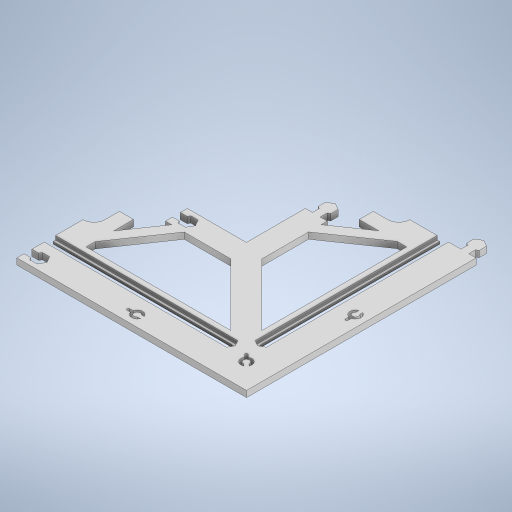
# Autodesk Inventor part: Vnejsi_ram
Saved by Autodesk Inventor 2024.2 (Build 282272000, 272)
## iProperties
Created: 2025-05-26
Part Number: Vnejsi_ram
Material: Všeobecné
Document SubType Name: Modeling
Designer: Elite
Density: 1 g/cm^3
Appearance: Výchozí
Author: Elite
Autodesk Inventor part; units mm, degrees
ref_plane "YZ Plane" through (0, 0, 0) normal (1, 0, 0) x (0, 1, 0)
ref_plane "XZ Plane" through (0, 0, 0) normal (0, 1, 0) x (-1, 0, 0)
ref_plane "XY Plane" through (0, 0, 0) normal (0, 0, 1) x (1, 0, 0)
sketch "Náčrt1" plane through (0, 0, 0) normal (0, 0, 1) x (1, 0, 0)
  line L0 (-41.907, -49.2472) -> (-39.5976, -53.2472)
  line L1 (-39.5976, -53.2472) -> (-41.907, -57.2472)
  line L2 (-41.907, -57.2472) -> (-46.5258, -57.2472)
  line L3 (-46.5258, -49.2472) -> (-41.907, -49.2472)
  line L4 (7.4742, -57.2472) -> (12.093, -57.2472)
  line L5 (12.093, -57.2472) -> (14.4024, -53.2472)
  line L6 (14.4024, -53.2472) -> (12.093, -49.2472)
  line L7 (12.093, -49.2472) -> (7.4742, -49.2472)
  line L8 (6.6082, -50.7472) -> (2.2836, -50.7472)
  line L9 (7.4742, -49.2472) -> (6.6082, -50.7472)
  line L10 (2.2836, -55.7472) -> (6.6082, -55.7472)
  line L11 (6.6082, -55.7472) -> (7.4742, -57.2472)
  line L12 (2.2836, -60.2472) -> (2.2836, -55.7472)
  line L13 (2.2836, -50.7472) -> (2.2836, -46.2472)
  line L14 (-17.7164, -60.2472) -> (2.2836, -60.2472)
  line L15 (2.2836, -46.2472) -> (-17.7164, -46.2472)
  line L16 (50.8236, 1.1022) -> (46.8236, 3.4116)
  line L17 (46.8236, 3.4116) -> (50.8236, 1.1022)
  line L18 (42.8236, 1.1022) -> (46.8236, 3.4116)
  line L19 (49.3236, -8.7072) -> (49.3236, -4.3826)
  line L20 (42.8236, -3.5166) -> (44.3236, -4.3826)
  line L21 (53.8236, -8.7072) -> (49.3236, -8.7072)
  line L22 (49.3236, -8.7072) -> (53.8236, -8.7072)
  line L23 (42.8236, 1.1022) -> (42.8236, -3.5166)
  line L24 (42.8236, -3.5166) -> (42.8236, 1.1022)
  line L25 (44.3236, -4.3826) -> (42.8236, -3.5166)
  line L26 (44.3236, -4.3826) -> (44.3236, -8.7072)
  line L27 (44.3236, -8.7072) -> (39.8236, -8.7072)
  line L28 (39.8236, -8.7072) -> (44.3236, -8.7072)
  line L29 (44.3236, -8.7072) -> (44.3236, -4.3826)
  line L30 (46.8236, 3.4116) -> (42.8236, 1.1022)
  line L31 (50.8236, -3.5166) -> (50.8236, 1.1022)
  line L32 (50.8236, 1.1022) -> (50.8236, -3.5166)
  line L33 (49.3236, -4.3826) -> (50.8236, -3.5166)
  line L34 (50.8236, -3.5166) -> (49.3236, -4.3826)
  line L35 (49.3236, -4.3826) -> (49.3236, -8.7072)
  line L36 (53.8236, 11.2928) -> (53.8236, -8.7072)
  line L37 (53.8236, -8.7072) -> (53.8236, 11.2928)
  line L38 (39.8236, -8.7072) -> (39.8236, 11.2928)
  line L39 (39.8236, 11.2928) -> (39.8236, -8.7072)
  line L40 (2.2836, -60.2472) -> (53.8236, -60.2472)
  line L41 (53.8236, -60.2472) -> (53.8236, -8.7072)
  line L42 (39.8236, -8.7072) -> (39.8236, -46.2472)
  line L43 (39.8236, -46.2472) -> (2.2836, -46.2472)
  arc A0 (-31.7164, -78.7074) -> (-17.7164, -78.7074) centre (-24.7164, -78.7074) ccw
  arc A1 (72.2839, 11.2928) -> (72.2839, 25.2928) centre (72.2839, 18.2928) ccw
  line L44 (53.8236, 11.2928) -> (72.2839, 11.2928)
  line L45 (72.2839, 25.2928) -> (53.8236, 25.2928)
  line L46 (-1.0283, -5.3953) -> (2.0296, -2.3374)
  line L47 (2.0296, -2.3374) -> (-1.0283, -5.3953)
  line L48 (2.0296, -2.3374) -> (3.7027, -2.7856)
  line L49 (3.7027, -2.7856) -> (2.0296, -2.3374)
  line L50 (3.5679, -9.9915) -> (-1.0283, -5.3953)
  line L51 (-1.0283, -5.3953) -> (3.5679, -9.9915)
  line L52 (-48.4045, -5.3953) -> (-53.0006, -9.9915)
  line L53 (-53.0006, -9.9915) -> (-48.4045, -5.3953)
  line L54 (-45.3465, -8.4532) -> (-48.4045, -5.3953)
  line L55 (-48.4045, -5.3953) -> (-45.3465, -8.4532)
  line L56 (-45.7948, -10.1263) -> (-45.3465, -8.4532)
  line L57 (-45.7948, -10.1263) -> (-42.5288, -13.3922)
  line L58 (-45.3465, -8.4532) -> (-45.7948, -10.1263)
  line L59 (-41.811, -4.9177) -> (-40.1379, -4.4694)
  line L60 (-40.1379, -4.4694) -> (-41.811, -4.9177)
  line L61 (-42.5288, -13.3922) -> (-45.7948, -10.1263)
  line L62 (-40.1379, -4.4694) -> (-36.872, -7.7354)
  line L63 (-36.872, -7.7354) -> (-40.1379, -4.4694)
  line L64 (-42.5288, -13.3922) -> (-38.0674, -12.1968)
  line L65 (-38.0674, -12.1968) -> (-36.872, -7.7354)
  line L66 (-36.872, -7.7354) -> (-38.0674, -12.1968)
  line L67 (-38.0674, -12.1968) -> (-42.5288, -13.3922)
  line L68 (-44.8689, -1.8598) -> (-41.811, -4.9177)
  line L69 (-41.811, -4.9177) -> (-44.8689, -1.8598)
  line L70 (-24.7164, -80.7891) -> (-28.3164, -78.7107)
  arc A2 (-26.7914, -76.5379) -> (-22.6414, -76.4898) centre (-24.715, -76.6291) ccw
  line L71 (-24.7164, -80.7891) -> (-28.3164, -78.7107)
  arc A3 (-31.7164, -78.7074) -> (-17.7164, -78.7074) centre (-24.7164, -78.7074) ccw
  arc A4 (-26.7914, -76.5379) -> (-22.6414, -76.4898) centre (-24.715, -76.6291) ccw
  line L72 (-21.1164, -78.7107) -> (-24.7164, -80.7891)
  line L73 (-21.1164, -78.7107) -> (-24.7164, -80.7891)
  line L74 (-31.7164, -60.2472) -> (-31.7164, -78.7074)
  line L75 (-31.7164, -78.7074) -> (-31.7164, -60.2472)
  line L76 (-17.7164, -60.2472) -> (-17.7164, -78.7074)
  line L77 (-17.7164, -78.7074) -> (-17.7164, -60.2472)
  line L78 (-41.907, -57.2472) -> (-39.5976, -53.2472)
  line L79 (-51.7164, -55.7472) -> (-47.3918, -55.7472)
  line L80 (-46.5258, -49.2472) -> (-47.3918, -50.7472)
  line L81 (-31.7164, -60.2472) -> (-51.7164, -60.2472)
  line L82 (-51.7164, -60.2472) -> (-31.7164, -60.2472)
  line L83 (-51.7164, -60.2472) -> (-51.7164, -55.7472)
  line L84 (-51.7164, -55.7472) -> (-51.7164, -60.2472)
  line L85 (-41.907, -49.2472) -> (-46.5258, -49.2472)
  line L86 (-47.3918, -50.7472) -> (-46.5258, -49.2472)
  line L87 (-51.7164, -46.2472) -> (-31.7164, -46.2472)
  line L88 (-31.7164, -46.2472) -> (-51.7164, -46.2472)
  line L89 (-47.3918, -50.7472) -> (-51.7164, -50.7472)
  line L90 (-51.7164, -50.7472) -> (-51.7164, -46.2472)
  line L91 (-51.7164, -46.2472) -> (-51.7164, -50.7472)
  line L92 (-51.7164, -50.7472) -> (-47.3918, -50.7472)
  line L93 (-26.7914, -29.9633) -> (-26.7914, -76.5379)
  line L94 (2.2836, -46.2472) -> (2.2836, -50.7472)
  line L95 (2.2836, -50.7472) -> (6.6082, -50.7472)
  line L96 (6.6082, -55.7472) -> (2.2836, -55.7472)
  line L97 (-24.7164, -25.7052) -> (-21.1164, -27.7837)
  line L98 (-28.3164, -27.7837) -> (-24.7164, -25.7052)
  line L99 (-17.7164, -21.0899) -> (-17.7164, -46.2472)
  arc A5 (-22.6414, -29.8845) -> (-26.7914, -29.9633) centre (-24.7175, -29.8628) ccw
  arc A6 (-53.0006, -9.9915) -> (-31.7164, -21.0899) centre (-24.7164, 18.2928) ccw
  arc A7 (-53.0006, -9.9915) -> (-31.7164, -21.0899) centre (-24.7164, 18.2928) ccw
  line L100 (-48.4045, -5.3953) -> (-45.3465, -8.4532)
  line L101 (-45.3465, -8.4532) -> (-48.4045, -5.3953)
  line L102 (-42.5288, -13.3922) -> (-38.0674, -12.1968)
  line L103 (-38.0674, -12.1968) -> (-42.5288, -13.3922)
  line L104 (-45.7948, -10.1263) -> (-42.5288, -13.3922)
  line L105 (-42.5288, -13.3922) -> (-45.7948, -10.1263)
  line L106 (-38.0674, -12.1968) -> (-36.872, -7.7354)
  line L107 (-36.872, -7.7354) -> (-38.0674, -12.1968)
  line L108 (-45.3465, -8.4532) -> (-45.7948, -10.1263)
  line L109 (-45.7948, -10.1263) -> (-45.3465, -8.4532)
  line L110 (-40.1379, -4.4694) -> (-36.872, -7.7354)
  line L111 (-36.872, -7.7354) -> (-40.1379, -4.4694)
  line L112 (-53.0006, -9.9915) -> (-48.4045, -5.3953)
  line L113 (-48.4045, -5.3953) -> (-53.0006, -9.9915)
  arc A8 (-17.7164, -21.0899) -> (3.5679, -9.9915) centre (-24.7164, 18.2928) ccw
  arc A9 (-17.7164, -21.0899) -> (3.5679, -9.9915) centre (-24.7164, 18.2928) ccw
  line L114 (-1.0283, -5.3953) -> (3.5679, -9.9915)
  line L115 (3.5679, -9.9915) -> (-1.0283, -5.3953)
  line L116 (2.0296, -2.3374) -> (-1.0283, -5.3953)
  line L117 (-1.0283, -5.3953) -> (2.0296, -2.3374)
  line L118 (3.7027, -2.7856) -> (2.0296, -2.3374)
  line L119 (2.0296, -2.3374) -> (3.7027, -2.7856)
  line L120 (-24.7164, -25.7052) -> (-21.1164, -27.7837)
  arc A10 (-22.6414, -29.8845) -> (-26.7914, -29.9633) centre (-24.7175, -29.8628) ccw
  line L121 (-28.3164, -27.7837) -> (-24.7164, -25.7052)
  line L122 (-17.7164, -46.2472) -> (-17.7164, -21.0899)
  line L123 (-31.7164, -46.2472) -> (-31.7164, -21.0899)
  line L124 (-31.7164, -21.0899) -> (-31.7164, -46.2472)
  line L125 (-39.5976, -53.2472) -> (-41.907, -49.2472)
  line L126 (-22.6414, -76.4898) -> (-22.6414, -29.8845)
  line L127 (-22.6414, -76.4898) -> (-22.6414, -29.8845)
  line L128 (-26.7914, -29.9633) -> (-26.7914, -76.5379)
  line L129 (-21.1164, -27.7837) -> (-21.1164, -78.7107)
  line L130 (-21.1164, -27.7837) -> (-21.1164, -78.7107)
  line L131 (-28.3164, -78.7107) -> (-28.3164, -27.7837)
  line L132 (-28.3164, -78.7107) -> (-28.3164, -27.7837)
  line L133 (-46.5258, -57.2472) -> (-41.907, -57.2472)
  line L134 (-47.3918, -55.7472) -> (-46.5258, -57.2472)
  line L135 (-46.5258, -57.2472) -> (-47.3918, -55.7472)
  line L136 (-47.3918, -55.7472) -> (-51.7164, -55.7472)
  line L137 (-40.1379, -4.4694) -> (-41.811, -4.9177)
  line L138 (-41.811, -4.9177) -> (-40.1379, -4.4694)
  line L139 (-41.811, -4.9177) -> (-44.8689, -1.8598)
  line L140 (-44.8689, -1.8598) -> (-41.811, -4.9177)
  line L141 (2.2836, -55.7472) -> (2.2836, -60.2472)
  line L142 (2.2836, -60.2472) -> (-17.7164, -60.2472)
  line L143 (-17.7164, -46.2472) -> (2.2836, -46.2472)
  line L144 (74.3655, 18.2928) -> (72.2871, 14.6928)
  arc A11 (70.1143, 16.2178) -> (70.0662, 20.3678) centre (70.2055, 18.2941) ccw
  line L145 (74.3655, 18.2928) -> (72.2871, 14.6928)
  arc A12 (72.2839, 11.2928) -> (72.2839, 25.2928) centre (72.2839, 18.2928) ccw
  arc A13 (70.1143, 16.2178) -> (70.0662, 20.3678) centre (70.2055, 18.2941) ccw
  line L146 (72.2871, 21.8928) -> (74.3655, 18.2928)
  line L147 (72.2871, 21.8928) -> (74.3655, 18.2928)
  line L148 (72.2839, 11.2928) -> (53.8236, 11.2928)
  line L149 (53.8236, 25.2928) -> (72.2839, 25.2928)
  line L150 (23.5397, 16.2178) -> (70.1143, 16.2178)
  line L151 (39.8236, 45.2928) -> (44.3236, 45.2928)
  line L152 (44.3236, 45.2928) -> (39.8236, 45.2928)
  line L153 (44.3236, 45.2928) -> (44.3236, 49.6174)
  line L154 (44.3236, 49.6174) -> (44.3236, 45.2928)
  line L155 (44.3236, 49.6174) -> (42.8236, 50.4834)
  line L156 (42.8236, 50.4834) -> (44.3236, 49.6174)
  line L157 (42.8236, 50.4834) -> (42.8236, 55.1022)
  line L158 (42.8236, 55.1022) -> (42.8236, 50.4834)
  line L159 (42.8236, 55.1022) -> (46.8236, 57.4116)
  line L160 (49.3236, 49.6174) -> (49.3236, 45.2928)
  line L161 (49.3236, 45.2928) -> (49.3236, 49.6174)
  line L162 (50.8236, 50.4834) -> (49.3236, 49.6174)
  line L163 (49.3236, 49.6174) -> (50.8236, 50.4834)
  line L164 (50.8236, 55.1022) -> (50.8236, 50.4834)
  line L165 (50.8236, 50.4834) -> (50.8236, 55.1022)
  line L166 (46.8236, 57.4116) -> (50.8236, 55.1022)
  line L167 (50.8236, 55.1022) -> (46.8236, 57.4116)
  line L168 (46.8236, 57.4116) -> (42.8236, 55.1022)
  line L169 (19.2816, 18.2928) -> (21.3601, 21.8928)
  line L170 (21.3601, 14.6928) -> (19.2816, 18.2928)
  line L171 (14.6664, 25.2928) -> (39.8236, 25.2928)
  arc A14 (23.4609, 20.3678) -> (23.5397, 16.2178) centre (23.4392, 18.2916) ccw
  arc A15 (3.5679, -9.9915) -> (14.6664, 11.2928) centre (-24.7164, 18.2928) ccw
  arc A16 (3.5679, -9.9915) -> (14.6664, 11.2928) centre (-24.7164, 18.2928) ccw
  line L172 (6.9687, 0.4803) -> (5.7732, 4.9418)
  line L173 (5.7732, 4.9418) -> (6.9687, 0.4803)
  line L174 (3.7027, -2.7856) -> (6.9687, 0.4803)
  line L175 (6.9687, 0.4803) -> (3.7027, -2.7856)
  line L176 (5.7732, 4.9418) -> (1.3118, 6.1372)
  line L177 (1.3118, 6.1372) -> (5.7732, 4.9418)
  line L178 (-1.9542, 2.8712) -> (1.3118, 6.1372)
  line L179 (1.3118, 6.1372) -> (-1.9542, 2.8712)
  arc A17 (14.6664, 25.2928) -> (3.5679, 46.5771) centre (-24.7164, 18.2928) ccw
  arc A18 (14.6664, 25.2928) -> (3.5679, 46.5771) centre (-24.7164, 18.2928) ccw
  line L180 (-1.0283, 41.9809) -> (3.5679, 46.5771)
  line L181 (3.5679, 46.5771) -> (-1.0283, 41.9809)
  line L182 (-4.0862, 45.0388) -> (-1.0283, 41.9809)
  line L183 (-1.0283, 41.9809) -> (-4.0862, 45.0388)
  line L184 (-3.6379, 46.7118) -> (-4.0862, 45.0388)
  line L185 (-3.6379, 46.7118) -> (-6.9039, 49.9778)
  line L186 (-4.0862, 45.0388) -> (-3.6379, 46.7118)
  line L187 (-7.6218, 41.5033) -> (-9.2948, 41.055)
  line L188 (-9.2948, 41.055) -> (-7.6218, 41.5033)
  line L189 (-6.9039, 49.9778) -> (-3.6379, 46.7118)
  line L190 (-9.2948, 41.055) -> (-12.5608, 44.321)
  line L191 (-12.5608, 44.321) -> (-9.2948, 41.055)
  line L192 (-6.9039, 49.9778) -> (-11.3654, 48.7824)
  line L193 (-11.3654, 48.7824) -> (-12.5608, 44.321)
  line L194 (-12.5608, 44.321) -> (-11.3654, 48.7824)
  line L195 (-11.3654, 48.7824) -> (-6.9039, 49.9778)
  line L196 (19.2816, 18.2928) -> (21.3601, 21.8928)
  arc A19 (23.4609, 20.3678) -> (23.5397, 16.2178) centre (23.4392, 18.2916) ccw
  line L197 (21.3601, 14.6928) -> (19.2816, 18.2928)
  line L198 (39.8236, 25.2928) -> (14.6664, 25.2928)
  line L199 (39.8236, 11.2928) -> (14.6664, 11.2928)
  line L200 (14.6664, 11.2928) -> (39.8236, 11.2928)
  line L201 (70.0662, 20.3678) -> (23.4609, 20.3678)
  line L202 (70.0662, 20.3678) -> (23.4609, 20.3678)
  line L203 (23.5397, 16.2178) -> (70.1143, 16.2178)
  line L204 (21.3601, 21.8928) -> (72.2871, 21.8928)
  line L205 (21.3601, 21.8928) -> (72.2871, 21.8928)
  line L206 (72.2871, 14.6928) -> (21.3601, 14.6928)
  line L207 (72.2871, 14.6928) -> (21.3601, 14.6928)
  line L208 (-1.9542, 2.8712) -> (-1.5059, 1.1982)
  line L209 (-1.5059, 1.1982) -> (-1.9542, 2.8712)
  line L210 (-1.5059, 1.1982) -> (-4.5638, -1.8598)
  line L211 (-4.5638, -1.8598) -> (-1.5059, 1.1982)
  line L212 (-4.5638, 38.4453) -> (-7.6218, 41.5033)
  line L213 (-7.6218, 41.5033) -> (-4.5638, 38.4453)
  line L214 (-4.5638, -1.8598) -> (-21.1808, 14.7573)
  line L215 (-21.1808, 14.7573) -> (-4.5638, -1.8598)
  arc A20 (-21.1808, 14.7573) -> (-21.1808, 21.8283) centre (-24.7164, 18.2928) ccw
  arc A21 (-21.1808, 14.7573) -> (-21.1808, 21.8283) centre (-24.7164, 18.2928) ccw
  line L216 (-4.5638, 38.4453) -> (-21.1808, 21.8283)
  line L217 (-21.1808, 21.8283) -> (-4.5638, 38.4453)
  line L218 (39.8236, 45.2928) -> (39.8236, 25.2928)
  line L219 (53.8236, 45.2928) -> (49.3236, 45.2928)
  line L220 (53.8236, 25.2928) -> (53.8236, 45.2928)
  line L221 (49.3236, 45.2928) -> (53.8236, 45.2928)
  line L222 (53.8236, 45.2928) -> (53.8236, 25.2928)
  line L223 (39.8236, 25.2928) -> (39.8236, 45.2928)
  line L224 (-24.7164, 117.3747) -> (-21.1164, 115.2962)
  arc A22 (-22.6414, 113.1234) -> (-26.7914, 113.0754) centre (-24.7177, 113.2147) ccw
  line L225 (-24.7164, 117.3747) -> (-21.1164, 115.2962)
  arc A23 (-17.7164, 115.293) -> (-31.7164, 115.293) centre (-24.7164, 115.293) ccw
  arc A24 (-17.7164, 115.293) -> (-31.7164, 115.293) centre (-24.7164, 115.293) ccw
  arc A25 (-22.6414, 113.1234) -> (-26.7914, 113.0754) centre (-24.7177, 113.2147) ccw
  line L226 (-28.3164, 115.2962) -> (-24.7164, 117.3747)
  line L227 (-28.3164, 115.2962) -> (-24.7164, 117.3747)
  line L228 (-17.7164, 96.8328) -> (-17.7164, 115.293)
  line L229 (-17.7164, 115.293) -> (-17.7164, 96.8328)
  line L230 (-31.7164, 96.8328) -> (-31.7164, 115.293)
  line L231 (-31.7164, 115.293) -> (-31.7164, 96.8328)
  line L232 (-7.5258, 93.8328) -> (-9.8352, 89.8328)
  line L233 (-9.8352, 89.8328) -> (-7.5258, 93.8328)
  line L234 (-7.5258, 85.8328) -> (-9.8352, 89.8328)
  line L235 (2.2836, 92.3328) -> (-2.0409, 92.3328)
  line L236 (-2.907, 85.8328) -> (-2.0409, 87.3328)
  line L237 (-17.7164, 96.8328) -> (2.2836, 96.8328)
  line L238 (2.2836, 96.8328) -> (-17.7164, 96.8328)
  line L239 (2.2836, 96.8328) -> (2.2836, 92.3328)
  line L240 (2.2836, 92.3328) -> (2.2836, 96.8328)
  line L241 (-7.5258, 85.8328) -> (-2.907, 85.8328)
  line L242 (-2.907, 85.8328) -> (-7.5258, 85.8328)
  line L243 (-2.0409, 87.3328) -> (-2.907, 85.8328)
  line L244 (2.2836, 82.8328) -> (-17.7164, 82.8328)
  line L245 (-17.7164, 82.8328) -> (2.2836, 82.8328)
  line L246 (-2.0409, 87.3328) -> (2.2836, 87.3328)
  line L247 (2.2836, 87.3328) -> (2.2836, 82.8328)
  line L248 (2.2836, 82.8328) -> (2.2836, 87.3328)
  line L249 (2.2836, 87.3328) -> (-2.0409, 87.3328)
  line L250 (-22.6414, 66.5489) -> (-22.6414, 113.1234)
  line L251 (-51.7164, 82.8328) -> (-51.7164, 87.3328)
  line L252 (-51.7164, 87.3328) -> (-51.7164, 82.8328)
  line L253 (-51.7164, 87.3328) -> (-56.0409, 87.3328)
  line L254 (-56.0409, 87.3328) -> (-51.7164, 87.3328)
  line L255 (-56.0409, 87.3328) -> (-56.907, 85.8328)
  line L256 (-56.907, 85.8328) -> (-56.0409, 87.3328)
  line L257 (-56.907, 85.8328) -> (-61.5258, 85.8328)
  line L258 (-61.5258, 85.8328) -> (-56.907, 85.8328)
  line L259 (-61.5258, 85.8328) -> (-63.8352, 89.8328)
  line L260 (-56.0409, 92.3328) -> (-51.7164, 92.3328)
  line L261 (-51.7164, 92.3328) -> (-56.0409, 92.3328)
  line L262 (-56.907, 93.8328) -> (-56.0409, 92.3328)
  line L263 (-56.0409, 92.3328) -> (-56.907, 93.8328)
  line L264 (-61.5258, 93.8328) -> (-56.907, 93.8328)
  line L265 (-56.907, 93.8328) -> (-61.5258, 93.8328)
  line L266 (-63.8352, 89.8328) -> (-61.5258, 93.8328)
  line L267 (-61.5258, 93.8328) -> (-63.8352, 89.8328)
  line L268 (-63.8352, 89.8328) -> (-61.5258, 85.8328)
  line L269 (-24.7164, 62.2908) -> (-28.3164, 64.3693)
  line L270 (-21.1164, 64.3693) -> (-24.7164, 62.2908)
  line L271 (-31.7164, 57.6755) -> (-31.7164, 82.8328)
  arc A26 (-26.7914, 66.47) -> (-22.6414, 66.5489) centre (-24.7152, 66.4483) ccw
  arc A27 (3.5679, 46.5771) -> (-17.7164, 57.6755) centre (-24.7164, 18.2928) ccw
  arc A28 (3.5679, 46.5771) -> (-17.7164, 57.6755) centre (-24.7164, 18.2928) ccw
  line L272 (-1.0283, 41.9809) -> (-4.0862, 45.0388)
  line L273 (-4.0862, 45.0388) -> (-1.0283, 41.9809)
  line L274 (-6.9039, 49.9778) -> (-11.3654, 48.7824)
  line L275 (-11.3654, 48.7824) -> (-6.9039, 49.9778)
  line L276 (-3.6379, 46.7118) -> (-6.9039, 49.9778)
  line L277 (-6.9039, 49.9778) -> (-3.6379, 46.7118)
  line L278 (-11.3654, 48.7824) -> (-12.5608, 44.321)
  line L279 (-12.5608, 44.321) -> (-11.3654, 48.7824)
  line L280 (-4.0862, 45.0388) -> (-3.6379, 46.7118)
  line L281 (-3.6379, 46.7118) -> (-4.0862, 45.0388)
  line L282 (-9.2948, 41.055) -> (-12.5608, 44.321)
  line L283 (-12.5608, 44.321) -> (-9.2948, 41.055)
  line L284 (3.5679, 46.5771) -> (-1.0283, 41.9809)
  line L285 (-1.0283, 41.9809) -> (3.5679, 46.5771)
  arc A29 (-31.7164, 57.6755) -> (-53.0006, 46.5771) centre (-24.7164, 18.2928) ccw
  arc A30 (-31.7164, 57.6755) -> (-53.0006, 46.5771) centre (-24.7164, 18.2928) ccw
  line L286 (-48.4045, 41.9809) -> (-53.0006, 46.5771)
  line L287 (-53.0006, 46.5771) -> (-48.4045, 41.9809)
  line L288 (-51.4624, 38.9229) -> (-48.4045, 41.9809)
  line L289 (-48.4045, 41.9809) -> (-51.4624, 38.9229)
  line L290 (-53.1354, 39.3712) -> (-51.4624, 38.9229)
  line L291 (-53.1354, 39.3712) -> (-56.4014, 36.1052)
  line L292 (-51.4624, 38.9229) -> (-53.1354, 39.3712)
  line L293 (-47.9269, 35.3874) -> (-47.4786, 33.7144)
  line L294 (-47.4786, 33.7144) -> (-47.9269, 35.3874)
  line L295 (-56.4014, 36.1052) -> (-53.1354, 39.3712)
  line L296 (-47.4786, 33.7144) -> (-50.7446, 30.4484)
  line L297 (-50.7446, 30.4484) -> (-47.4786, 33.7144)
  line L298 (-56.4014, 36.1052) -> (-55.206, 31.6438)
  line L299 (-55.206, 31.6438) -> (-50.7446, 30.4484)
  line L300 (-50.7446, 30.4484) -> (-55.206, 31.6438)
  line L301 (-55.206, 31.6438) -> (-56.4014, 36.1052)
  line L302 (-24.7164, 62.2908) -> (-28.3164, 64.3693)
  arc A31 (-26.7914, 66.47) -> (-22.6414, 66.5489) centre (-24.7152, 66.4483) ccw
  line L303 (-21.1164, 64.3693) -> (-24.7164, 62.2908)
  line L304 (-31.7164, 82.8328) -> (-31.7164, 57.6755)
  line L305 (-17.7164, 82.8328) -> (-17.7164, 57.6755)
  line L306 (-17.7164, 57.6755) -> (-17.7164, 82.8328)
  line L307 (-9.8352, 89.8328) -> (-7.5258, 85.8328)
  line L308 (-26.7914, 113.0754) -> (-26.7914, 66.47)
  line L309 (-26.7914, 113.0754) -> (-26.7914, 66.47)
  line L310 (-22.6414, 66.5489) -> (-22.6414, 113.1234)
  line L311 (-28.3164, 64.3693) -> (-28.3164, 115.2962)
  line L312 (-28.3164, 64.3693) -> (-28.3164, 115.2962)
  line L313 (-21.1164, 115.2962) -> (-21.1164, 64.3693)
  line L314 (-21.1164, 115.2962) -> (-21.1164, 64.3693)
  line L315 (-2.907, 93.8328) -> (-7.5258, 93.8328)
  line L316 (-7.5258, 93.8328) -> (-2.907, 93.8328)
  line L317 (-2.0409, 92.3328) -> (-2.907, 93.8328)
  line L318 (-2.907, 93.8328) -> (-2.0409, 92.3328)
  line L319 (-2.0409, 92.3328) -> (2.2836, 92.3328)
  line L320 (-9.2948, 41.055) -> (-7.6218, 41.5033)
  line L321 (-7.6218, 41.5033) -> (-9.2948, 41.055)
  line L322 (-7.6218, 41.5033) -> (-4.5638, 38.4453)
  line L323 (-4.5638, 38.4453) -> (-7.6218, 41.5033)
  line L324 (-44.8689, 38.4453) -> (-47.9269, 35.3874)
  line L325 (-47.9269, 35.3874) -> (-44.8689, 38.4453)
  line L326 (-4.5638, 38.4453) -> (-21.1808, 21.8283)
  line L327 (-21.1808, 21.8283) -> (-4.5638, 38.4453)
  arc A32 (-21.1808, 21.8283) -> (-28.2519, 21.8283) centre (-24.7164, 18.2928) ccw
  arc A33 (-21.1808, 21.8283) -> (-28.2519, 21.8283) centre (-24.7164, 18.2928) ccw
  line L328 (-44.8689, 38.4453) -> (-28.2519, 21.8283)
  line L329 (-28.2519, 21.8283) -> (-44.8689, 38.4453)
  line L330 (-51.7164, 82.8328) -> (-31.7164, 82.8328)
  line L331 (-51.7164, 96.8328) -> (-51.7164, 92.3328)
  line L332 (-31.7164, 96.8328) -> (-51.7164, 96.8328)
  line L333 (-51.7164, 92.3328) -> (-51.7164, 96.8328)
  line L334 (-51.7164, 96.8328) -> (-31.7164, 96.8328)
  line L335 (-31.7164, 82.8328) -> (-51.7164, 82.8328)
  line L336 (-123.7983, 18.2928) -> (-121.7198, 21.8928)
  arc A34 (-119.547, 20.3678) -> (-119.499, 16.2178) centre (-119.6383, 18.2915) ccw
  line L337 (-123.7983, 18.2928) -> (-121.7198, 21.8928)
  arc A35 (-121.7166, 25.2928) -> (-121.7166, 11.2928) centre (-121.7166, 18.2928) ccw
  arc A36 (-121.7166, 25.2928) -> (-121.7166, 11.2928) centre (-121.7166, 18.2928) ccw
  arc A37 (-119.547, 20.3678) -> (-119.499, 16.2178) centre (-119.6383, 18.2915) ccw
  line L338 (-121.7198, 14.6928) -> (-123.7983, 18.2928)
  line L339 (-121.7198, 14.6928) -> (-123.7983, 18.2928)
  line L340 (-103.2563, 25.2928) -> (-121.7166, 25.2928)
  line L341 (-121.7166, 25.2928) -> (-103.2563, 25.2928)
  line L342 (-103.2563, 11.2928) -> (-121.7166, 11.2928)
  line L343 (-121.7166, 11.2928) -> (-103.2563, 11.2928)
  line L344 (-100.2563, 35.4834) -> (-96.2563, 33.174)
  line L345 (-96.2563, 33.174) -> (-100.2563, 35.4834)
  line L346 (-92.2563, 35.4834) -> (-96.2563, 33.174)
  line L347 (-98.7563, 45.2928) -> (-98.7563, 40.9682)
  line L348 (-92.2563, 40.1022) -> (-93.7563, 40.9682)
  line L349 (-103.2563, 25.2928) -> (-103.2563, 45.2928)
  line L350 (-103.2563, 45.2928) -> (-103.2563, 25.2928)
  line L351 (-103.2563, 45.2928) -> (-98.7563, 45.2928)
  line L352 (-98.7563, 45.2928) -> (-103.2563, 45.2928)
  line L353 (-92.2563, 35.4834) -> (-92.2563, 40.1022)
  line L354 (-92.2563, 40.1022) -> (-92.2563, 35.4834)
  line L355 (-93.7563, 40.9682) -> (-92.2563, 40.1022)
  line L356 (-89.2563, 45.2928) -> (-89.2563, 25.2928)
  line L357 (-89.2563, 25.2928) -> (-89.2563, 45.2928)
  line L358 (-93.7563, 40.9682) -> (-93.7563, 45.2928)
  line L359 (-93.7563, 45.2928) -> (-89.2563, 45.2928)
  line L360 (-89.2563, 45.2928) -> (-93.7563, 45.2928)
  line L361 (-93.7563, 45.2928) -> (-93.7563, 40.9682)
  line L362 (-72.9724, 20.3678) -> (-119.547, 20.3678)
  line L363 (-89.2563, -8.7072) -> (-93.7563, -8.7072)
  line L364 (-93.7563, -8.7072) -> (-89.2563, -8.7072)
  line L365 (-93.7563, -8.7072) -> (-93.7563, -13.0318)
  line L366 (-93.7563, -13.0318) -> (-93.7563, -8.7072)
  line L367 (-93.7563, -13.0318) -> (-92.2563, -13.8978)
  line L368 (-92.2563, -13.8978) -> (-93.7563, -13.0318)
  line L369 (-92.2563, -13.8978) -> (-92.2563, -18.5166)
  line L370 (-92.2563, -18.5166) -> (-92.2563, -13.8978)
  line L371 (-92.2563, -18.5166) -> (-96.2563, -20.826)
  line L372 (-98.7563, -13.0318) -> (-98.7563, -8.7072)
  line L373 (-98.7563, -8.7072) -> (-98.7563, -13.0318)
  line L374 (-100.2563, -13.8978) -> (-98.7563, -13.0318)
  line L375 (-98.7563, -13.0318) -> (-100.2563, -13.8978)
  line L376 (-100.2563, -18.5166) -> (-100.2563, -13.8978)
  line L377 (-100.2563, -13.8978) -> (-100.2563, -18.5166)
  line L378 (-96.2563, -20.826) -> (-100.2563, -18.5166)
  line L379 (-100.2563, -18.5166) -> (-96.2563, -20.826)
  line L380 (-96.2563, -20.826) -> (-92.2563, -18.5166)
  line L381 (-68.7144, 18.2928) -> (-70.7928, 14.6928)
  line L382 (-70.7928, 21.8928) -> (-68.7144, 18.2928)
  line L383 (-64.0991, 11.2928) -> (-89.2563, 11.2928)
  arc A38 (-72.8936, 16.2178) -> (-72.9724, 20.3678) centre (-72.8719, 18.294) ccw
  arc A39 (-53.0006, 46.5771) -> (-64.0991, 25.2928) centre (-24.7164, 18.2928) ccw
  arc A40 (-53.0006, 46.5771) -> (-64.0991, 25.2928) centre (-24.7164, 18.2928) ccw
  line L384 (-48.4045, 41.9809) -> (-51.4624, 38.9229)
  line L385 (-51.4624, 38.9229) -> (-48.4045, 41.9809)
  line L386 (-56.4014, 36.1052) -> (-55.206, 31.6438)
  line L387 (-55.206, 31.6438) -> (-56.4014, 36.1052)
  line L388 (-53.1354, 39.3712) -> (-56.4014, 36.1052)
  line L389 (-56.4014, 36.1052) -> (-53.1354, 39.3712)
  line L390 (-55.206, 31.6438) -> (-50.7446, 30.4484)
  line L391 (-50.7446, 30.4484) -> (-55.206, 31.6438)
  line L392 (-51.4624, 38.9229) -> (-53.1354, 39.3712)
  line L393 (-53.1354, 39.3712) -> (-51.4624, 38.9229)
  line L394 (-47.4786, 33.7144) -> (-50.7446, 30.4484)
  line L395 (-50.7446, 30.4484) -> (-47.4786, 33.7144)
  line L396 (-53.0006, 46.5771) -> (-48.4045, 41.9809)
  line L397 (-48.4045, 41.9809) -> (-53.0006, 46.5771)
  arc A41 (-64.0991, 11.2928) -> (-53.0006, -9.9915) centre (-24.7164, 18.2928) ccw
  arc A42 (-64.0991, 11.2928) -> (-53.0006, -9.9915) centre (-24.7164, 18.2928) ccw
  line L398 (-68.7144, 18.2928) -> (-70.7928, 14.6928)
  arc A43 (-72.8936, 16.2178) -> (-72.9724, 20.3678) centre (-72.8719, 18.294) ccw
  line L399 (-70.7928, 21.8928) -> (-68.7144, 18.2928)
  line L400 (-89.2563, 11.2928) -> (-64.0991, 11.2928)
  line L401 (-89.2563, 25.2928) -> (-64.0991, 25.2928)
  line L402 (-64.0991, 25.2928) -> (-89.2563, 25.2928)
  line L403 (-96.2563, 33.174) -> (-92.2563, 35.4834)
  line L404 (-119.499, 16.2178) -> (-72.8936, 16.2178)
  line L405 (-119.499, 16.2178) -> (-72.8936, 16.2178)
  line L406 (-72.9724, 20.3678) -> (-119.547, 20.3678)
  line L407 (-70.7928, 14.6928) -> (-121.7198, 14.6928)
  line L408 (-70.7928, 14.6928) -> (-121.7198, 14.6928)
  line L409 (-121.7198, 21.8928) -> (-70.7928, 21.8928)
  line L410 (-121.7198, 21.8928) -> (-70.7928, 21.8928)
  line L411 (-100.2563, 40.1022) -> (-100.2563, 35.4834)
  line L412 (-100.2563, 35.4834) -> (-100.2563, 40.1022)
  line L413 (-98.7563, 40.9682) -> (-100.2563, 40.1022)
  line L414 (-100.2563, 40.1022) -> (-98.7563, 40.9682)
  line L415 (-98.7563, 40.9682) -> (-98.7563, 45.2928)
  line L416 (-47.4786, 33.7144) -> (-47.9269, 35.3874)
  line L417 (-47.9269, 35.3874) -> (-47.4786, 33.7144)
  line L418 (-47.9269, 35.3874) -> (-44.8689, 38.4453)
  line L419 (-44.8689, 38.4453) -> (-47.9269, 35.3874)
  line L420 (-44.8689, 38.4453) -> (-28.2519, 21.8283)
  line L421 (-28.2519, 21.8283) -> (-44.8689, 38.4453)
  arc A44 (-28.2519, 21.8283) -> (-28.2519, 14.7573) centre (-24.7164, 18.2928) ccw
  arc A45 (-28.2519, 21.8283) -> (-28.2519, 14.7573) centre (-24.7164, 18.2928) ccw
  line L422 (-44.8689, -1.8598) -> (-28.2519, 14.7573)
  line L423 (-28.2519, 14.7573) -> (-44.8689, -1.8598)
  line L424 (-89.2563, -8.7072) -> (-89.2563, 11.2928)
  line L425 (-103.2563, -8.7072) -> (-98.7563, -8.7072)
  line L426 (-103.2563, 11.2928) -> (-103.2563, -8.7072)
  line L427 (-98.7563, -8.7072) -> (-103.2563, -8.7072)
  line L428 (-103.2563, -8.7072) -> (-103.2563, 11.2928)
  line L429 (-89.2563, 11.2928) -> (-89.2563, -8.7072)
  line L430 (3.7027, -2.7856) -> (6.9687, 0.4803)
  line L431 (-1.5059, 1.1982) -> (-1.9542, 2.8712)
  line L432 (-1.9542, 2.8712) -> (-1.5059, 1.1982)
  line L433 (6.9687, 0.4803) -> (3.7027, -2.7856)
  line L434 (-1.9542, 2.8712) -> (1.3118, 6.1372)
  line L435 (1.3118, 6.1372) -> (-1.9542, 2.8712)
  line L436 (6.9687, 0.4803) -> (5.7732, 4.9418)
  line L437 (5.7732, 4.9418) -> (1.3118, 6.1372)
  line L438 (1.3118, 6.1372) -> (5.7732, 4.9418)
  line L439 (5.7732, 4.9418) -> (6.9687, 0.4803)
  line L440 (-4.5638, -1.8598) -> (-1.5059, 1.1982)
  line L441 (-1.5059, 1.1982) -> (-4.5638, -1.8598)
  line L442 (-44.8689, -1.8598) -> (-28.2519, 14.7573)
  line L443 (-28.2519, 14.7573) -> (-44.8689, -1.8598)
  arc A46 (-28.2519, 14.7573) -> (-21.1808, 14.7573) centre (-24.7164, 18.2928) ccw
  arc A47 (-28.2519, 14.7573) -> (-21.1808, 14.7573) centre (-24.7164, 18.2928) ccw
  line L444 (-4.5638, -1.8598) -> (-21.1808, 14.7573)
  line L445 (-21.1808, 14.7573) -> (-4.5638, -1.8598)
  line L446 (-24.7164, -85.7074) -> (-24.7164, -99.7074)
  line L447 (-24.7164, -99.7074) -> (93.2839, -99.7074)
  line L448 (93.2839, 18.2945) -> (93.2839, -99.7074)
  line L449 (-24.7164, -99.7074) -> (-24.7164, -113.7074)
  line L450 (-24.7164, -99.7074) -> (-10.7164, -99.7074) construction
  line L451 (-24.7164, -113.7074) -> (107.4113, -113.7074)
  line L452 (107.4113, -113.7074) -> (107.4113, 18.2945)
  line L453 (93.2839, -99.7074) -> (53.8236, -60.2472)
  line L454 (83.3844, -99.7074) -> (43.9241, -60.2472)
  line L455 (93.2839, -89.8079) -> (53.8236, -50.3477)
  line L456 (114.2839, 18.2928) -> (111.7839, 18.2928)
  line L457 (114.2839, 18.2928) -> (116.7839, 18.2928)
  line L458 (111.7839, 18.2928) -> (111.7839, 21.7928)
  line L459 (116.7839, 21.7928) -> (116.7839, 18.2928)
  line L460 (111.7839, 21.7928) -> (116.7839, 21.7928)
  line L461 (111.7839, 21.7928) -> (111.7839, 22.6174)
  line L462 (116.7839, 21.7928) -> (116.7839, 22.6174)
  line L463 (111.7839, 22.6174) -> (110.2839, 23.4834)
  line L464 (118.2839, 23.4834) -> (116.7839, 22.6174)
  line L465 (110.2839, 23.4834) -> (110.2839, 28.1022)
  line L466 (110.2839, 28.1022) -> (114.2839, 30.4116)
  line L467 (114.2839, 30.4116) -> (118.2839, 28.1022)
  line L468 (118.2839, 28.1022) -> (118.2839, 23.4834)
  line L469 (107.4113, 18.2945) -> (93.2839, 18.2945)
  line L470 (107.4113, 18.2945) -> (114.4113, 18.2929)
  line L471 (114.4113, 18.2929) -> (114.4113, 4.2929)
  line L472 (114.4113, 4.2929) -> (121.4113, 4.2929)
  line L473 (121.4113, 4.2929) -> (121.4113, 18.2928)
  line L474 (121.4113, 18.2928) -> (116.7839, 18.2928)
  line L475 (114.4113, 4.2929) -> (107.4113, 4.2929)
  line L476 (-19.5258, -124.7074) -> (-14.907, -124.7074)
  line L477 (-14.907, -124.7074) -> (-12.5976, -120.7074)
  line L478 (-20.3918, -118.2074) -> (-24.7164, -118.2074)
  line L479 (-24.7164, -123.2074) -> (-20.3918, -123.2074)
  line L480 (-20.3918, -123.2074) -> (-19.5258, -124.7074)
  line L481 (-24.7164, -127.7074) -> (-24.7164, -123.2074)
  line L482 (-12.5976, -120.7074) -> (-14.907, -116.7074)
  line L483 (-14.907, -116.7074) -> (-19.5258, -116.7074)
  line L484 (-19.5258, -116.7074) -> (-20.3918, -118.2074)
  line L485 (-24.7164, -118.2074) -> (-24.7164, -113.7074)
  line L486 (-20.3918, -123.2074) -> (-24.7164, -123.2074)
  line L487 (-24.7164, -118.2074) -> (-20.3918, -118.2074)
  line L488 (-24.7164, -113.7074) -> (-24.7164, -118.2074)
  line L489 (-24.7164, -123.2074) -> (-24.7164, -127.7074)
  line L490 (-24.7164, -127.7074) -> (0.2836, -127.7074)
  line L491 (0.2836, -127.7074) -> (0.2836, -113.7074)
  line L492 (93.2839, -99.7074) -> (93.2839, -113.7074)
  line L493 (93.2839, -106.7074) -> (107.4113, -106.7074)
  line L494 (93.2839, -106.7074) -> (91.2054, -110.3074)
  line L495 (-24.7164, -108.7824) -> (89.0963, -108.7824)
  line L496 (93.2839, -106.7074) -> (91.2054, -110.3074)
  line L497 (89.0483, -104.6324) -> (-24.7164, -104.6324)
  line L498 (42.5217, -108.7824) -> (89.0963, -108.7824)
  line L499 (91.2054, -110.3074) -> (-24.7164, -110.3074)
  line L500 (91.2054, -110.3074) -> (40.2784, -110.3074)
  arc A48 (89.0963, -108.7824) -> (89.0483, -104.6324) centre (89.1875, -106.7061) ccw
  arc A49 (89.0963, -108.7824) -> (89.0483, -104.6324) centre (89.1875, -106.7061) ccw
  line L501 (91.2054, -103.1074) -> (93.2839, -106.7074)
  line L502 (91.2054, -103.1074) -> (93.2839, -106.7074)
  line L503 (89.0483, -104.6324) -> (42.4429, -104.6324)
  line L504 (91.2054, -103.1074) -> (-24.7164, -103.1074)
  line L505 (100.3476, -106.7074) -> (100.3476, -109.7654)
  line L506 (102.4226, -95.4081) -> (102.4226, -48.8028)
  line L507 (98.2726, -48.8816) -> (98.2726, -95.4562)
  arc A50 (98.2726, -95.4562) -> (102.4226, -95.4081) centre (100.3489, -95.5474) ccw
  arc A51 (98.2726, -95.4562) -> (102.4226, -95.4081) centre (100.3489, -95.5474) ccw
  line L508 (96.7476, -97.5653) -> (96.7476, -46.6383)
  line L509 (102.4226, -95.4081) -> (102.4226, 18.3565)
  line L510 (98.2726, 18.3565) -> (98.2726, -95.4562)
  line L511 (103.9476, -97.5653) -> (103.9476, 18.3565)
  line L512 (96.7476, -97.5653) -> (96.7476, 18.3565)
  line L513 (103.9476, -97.5653) -> (100.3476, -99.6437)
  line L514 (103.9476, -97.5653) -> (100.3476, -99.6437)
  line L515 (100.3476, -99.6437) -> (96.7476, -97.5653)
  line L516 (100.3476, -99.6437) -> (96.7476, -97.5653)
  line L517 (-17.7164, -69.4773) -> (-8.7164, -69.4773)
  line L518 (-8.7164, -69.4773) -> (-8.7164, -99.7074)
  line L519 (63.0537, 11.2928) -> (63.0537, 2.2928)
  line L520 (63.0537, 2.2928) -> (93.2839, 2.2928)
  line L521 (79.2839, 18.2928) -> (93.2839, 18.2872)
  line L522 (-8.7164, -99.7074) -> (-8.7164, -95.7074)
  line L523 (0.2836, -127.7074) -> (107.4113, -127.7074)
  line L524 (107.4113, -127.7074) -> (121.4113, -127.7074)
  line L525 (121.4113, -127.7074) -> (121.4113, 4.2929)
  line L526 (-8.7164, -95.7074) -> (79.3844, -95.7074)
  line L527 (93.2839, 2.2928) -> (89.2839, 2.2928)
  line L528 (89.2839, 2.2928) -> (89.2839, -85.8079)
  point P0 (0, 0)
  point P1 (114.2839, 21.7928)
  point P2 (114.2839, 25.7928)
  point P3 (111.7839, 18.2935)
  point P4 (91.2022, -106.7074)
  point P5 (91.2022, -106.7074)
  point P6 (100.3476, -97.562)
  point P7 (100.3476, -97.562)
  point P8 (103.9476, 18.2945)
  point P9 (102.4226, 18.2945)
  point P10 (98.2726, 18.2945)
  point P11 (96.7476, 18.2945)
  dimension "d0" = 14
  dimension "d1" = 14
  dimension "d2" = 14
  dimension "d4" = 7
  dimension "d5" = 7
  dimension "d6" = 3.5
  dimension "d7" = 5
  dimension "d8" = 8
  dimension "d9" = 4
  dimension "d14" = 7
  dimension "d15" = 14
  dimension "d16" = 7
  dimension "d17" = 25
  dimension "d18" = 14
  dimension "d24" = 90
  dimension "d36" = 30.2301
  dimension "d37" = 9
  dimension "d38" = 9
  dimension "d39" = 4
  dimension "d42" = 14
  dimension "d43" = 4
  dimension "d46" = 14
  dimension "d47" = 4.15
  constraints: 1058 end point, 106 point on circle, 52 centre point, 28 point on line, 15 perpendicular, 10 horizontal, 6 vertical, 5 midpoint, 2 parallel, 41 other
  measures "d0" distance of L446.start L447.start
  measures "d1" distance between parallel lines of L447 L451
  measures "d2" distance from line of L517.start L74
  measures "d4" distance between parallel lines of L453 L454
  measures "d5" distance between parallel lines of L453 L455
  measures "d6" distance of L458.start L461.start
  measures "d7" distance of L461.start L462.start
  measures "d8" distance between parallel lines of L468 L465
  measures "d9" distance of point (114.284, 21.793) point (114.284, 25.793)
  measures "d14" distance of L470.end L469.start
  measures "d15" distance of L470.end L471.end
  measures "d16" distance of L471.end L472.end
  measures "d17" distance of L490.start L490.end
  measures "d18" distance between parallel lines of L451 L490
  measures "d36" distance between parallel lines of L450 L517
  measures "d37" distance of L517.start L517.end
  measures "d38" distance of L519.start L519.end
  measures "d39" distance of L518.end L522.end
  measures "d42" distance of L523.end L524.end
  measures "d43" distance of L520.end L527.end
  measures "d46" distance between parallel lines of L148 L149
  measures "d47" distance between parallel lines of L150 L201
extrude "Vysunutí1" add sketch "Náčrt1" against normal blind 4 contours A0 L76 L517 L518 L447 L446 | L447 L492 L501 L504 L449 | L504 L501 L494 L499 L449 L495 A48 L497 | L454 L40 L453 L447 | L497 A48 L495 L449 | L12 L10 L11 L4 L5 L6 L7 L9 L8 L13 L43 L42 L27 L26 L20 L23 L18 L16 L31 L33 L19 L21 L41 L40 | L453 L41 L455 L448 | L448 L469 L512 L508 L515 L513 L511 L452 L493 L492 | L493 L452 L451 L492 | L492 L451 L449 L499 L494 | L451 L452 L475 L472 L525 L524 L523 L491 | L520 L519 L44 A1 L521 L448 | L451 L491 L490 L481 L479 L480 L476 L477 L482 L483 L484 L478 L485 | L452 L470 L456 L457 L471 L475 | L471 L457 L474 L473 L472 | L469 L510 L507 A50 L506 L509 L511 L513 L515 L508 L512 | L458 L460 L459 L457 L456 | L469 L509 L506 A50 L507 L510 | L461 L463 L465 L466 L467 L468 L464 L462 L460
sketch "Náčrt2" plane through (0, 0, -4) normal (0, 0, -1) x (1, 0, 0)
  line L0 (-24.7164, 99.7074) -> (-20.7164, 99.7074)
  line L1 (6.2836, 60.2472) -> (-20.7164, 99.7074)
  line L2 (6.2836, 60.2472) -> (14.2836, 60.2472)
  line L3 (-20.7164, 99.7074) -> (-12.7164, 99.7074)
  line L4 (-12.7164, 99.7074) -> (14.2836, 60.2472)
  line L5 (6.2836, 60.2472) -> (14.2836, 60.2472)
  line L6 (-12.7164, 99.7074) -> (-20.7164, 99.7074)
  line L7 (2.2836, 46.2472) -> (39.8236, 46.2472) projected
  line L8 (107.4113, 113.7074) -> (39.8236, 46.2472)
  line L9 (39.8236, 46.2472) -> (107.4113, 113.7074)
  line L10 (93.162, -18.3936) -> (93.1695, -14.3936)
  line L11 (53.7603, 12.6809) -> (93.1695, -14.3936)
  line L12 (53.7603, 12.6809) -> (53.7754, 20.6808)
  line L13 (93.1695, -14.3936) -> (93.1846, -6.3936)
  line L14 (93.1846, -6.3936) -> (53.7754, 20.6808)
  line L15 (53.7603, 12.6809) -> (53.7754, 20.6808)
  line L16 (93.1846, -6.3936) -> (93.1695, -14.3936)
  point P0 (0, 0)
  point P1 (2.2836, 60.2472)
  point P2 (53.7527, 8.6809)
  dimension "d30" = 4
  dimension "d31" = 4
  dimension "d32" = 8
  dimension "d33" = 8
  constraints: 32 end point, 6 symmetric about line, 2 collinear
  measures "d30" distance of L0.start L0.end
  measures "d31" distance of point (2.284, 60.247) L1.start
  measures "d32" distance of L1.start L2.end
  measures "d33" distance of L0.end L3.end
extrude "Vysunutí2" cut sketch "Náčrt1" against normal blind 2.5 contours L504 L501 L494 L499 L449 L495 A48 L497 | L469 L510 L507 A50 L506 L509 L511 L513 L515 L508 L512
extrude "Vysunutí3" cut sketch "Náčrt1" against normal through all contours L497 A48 L495 L449 | L469 L509 L506 A50 L507 L510
extrude "Vysunutí4" add sketch "Náčrt2" against normal blind 4
sketch "Náčrt3" plane through (0, 0, 0) normal (0, 0, 1) x (1, 0, 0)
  circle A0 centre (114.2839, -51.2073) radius 2
  circle A1 centre (114.2839, -51.2073) radius 3.5412
  circle A2 centre (114.2838, -56.8073) radius 0.85
  line L0 (113.4338, -56.8073) -> (113.4338, -54.645)
  line L1 (115.1339, -56.8073) -> (115.1339, -54.645)
  line L2 (113.0839, -49.6073) -> (113.0839, -47.8757)
  line L3 (115.4839, -49.6073) -> (115.4839, -47.8757)
  circle A3 centre (105.5498, -111.9415) radius 2
  circle A4 centre (105.5498, -111.9415) radius 3.5412
  circle A5 centre (101.59, -107.9817) radius 0.85
  line L4 (102.191, -107.3807) -> (103.72, -108.9097)
  line L5 (100.9889, -108.5828) -> (102.5179, -110.1118)
  line L6 (107.5297, -112.2243) -> (108.7542, -113.4488)
  line L7 (105.8326, -113.9214) -> (107.0571, -115.1459)
  line L8 (-8.7164, -82.1695) -> (-8.7164, -69.4773) projected
  line L9 (-8.7164, -69.4773) -> (-17.7164, -69.4773) projected
  line L10 (-17.7164, -69.4773) -> (-17.7164, -78.7074) projected
  arc A6 (-24.7164, -85.7074) -> (-17.7164, -78.7074) centre (-24.7164, -78.7074) ccw projected
  line L11 (-24.7164, -85.7074) -> (-24.7164, -103.1074) projected
  line L12 (-24.7164, -103.1074) -> (91.2054, -103.1074) projected
  line L13 (91.2054, -103.1074) -> (93.2839, -106.7074) projected
  line L14 (93.2839, -106.7074) -> (91.2054, -110.3074) projected
  line L15 (91.2054, -110.3074) -> (-24.7164, -110.3074) projected
  line L16 (-24.7164, -110.3074) -> (-24.7164, -118.2074) projected
  line L17 (-24.7164, -118.2074) -> (-20.3918, -118.2074) projected
  line L18 (-20.3918, -118.2074) -> (-19.5258, -116.7074) projected
  line L19 (-19.5258, -116.7074) -> (-14.907, -116.7074) projected
  line L20 (-14.907, -116.7074) -> (-12.5976, -120.7074) projected
  line L21 (-12.5976, -120.7074) -> (-14.907, -124.7074) projected
  line L22 (-14.907, -124.7074) -> (-19.5258, -124.7074) projected
  line L23 (-19.5258, -124.7074) -> (-20.3918, -123.2074) projected
  line L24 (-20.3918, -123.2074) -> (-24.7164, -123.2074) projected
  line L25 (-24.7164, -123.2074) -> (-24.7164, -127.7074) projected
  line L26 (-24.7164, -127.7074) -> (121.4113, -127.7074) projected
  line L27 (121.4113, -127.7074) -> (121.4113, 18.2928) projected
  line L28 (121.4113, 18.2928) -> (116.7839, 18.2928) projected
  line L29 (116.7839, 18.2928) -> (116.7839, 22.6174) projected
  line L30 (116.7839, 22.6174) -> (118.2839, 23.4834) projected
  line L31 (118.2839, 23.4834) -> (118.2839, 28.1022) projected
  line L32 (118.2839, 28.1022) -> (114.2839, 30.4116) projected
  line L33 (114.2839, 30.4116) -> (110.2839, 28.1022) projected
  line L34 (110.2839, 28.1022) -> (110.2839, 23.4834) projected
  line L35 (110.2839, 23.4834) -> (111.7839, 22.6174) projected
  line L36 (111.7839, 22.6174) -> (111.7839, 18.2935) projected
  line L37 (111.7839, 18.2935) -> (107.4113, 18.2945) projected
  line L38 (107.4113, 18.2945) -> (103.9476, 18.2945) projected
  line L39 (103.9476, 18.2945) -> (103.9476, -97.5653) projected
  line L40 (103.9476, -97.5653) -> (100.3476, -99.6437) projected
  line L41 (100.3476, -99.6437) -> (96.7476, -97.5653) projected
  line L42 (96.7476, -97.5653) -> (96.7476, 18.2945) projected
  line L43 (96.7476, 18.2945) -> (93.2839, 18.2945) projected
  line L44 (93.2839, 18.2945) -> (93.2839, 18.2872) projected
  line L45 (93.2839, 18.2872) -> (79.2839, 18.2928) projected
  arc A7 (72.2839, 11.2928) -> (79.2839, 18.2928) centre (72.2839, 18.2928) ccw projected
  line L46 (72.2839, 11.2928) -> (63.0537, 11.2928) projected
  line L47 (63.0537, 11.2928) -> (63.0537, 2.2928) projected
  line L48 (63.0537, 2.2928) -> (75.5558, 2.2928) projected
  line L49 (75.5558, 2.2928) -> (53.8236, -12.6374) projected
  line L50 (53.8236, -12.6374) -> (53.8236, -8.7072) projected
  line L51 (53.8236, -8.7072) -> (49.3236, -8.7072) projected
  line L52 (49.3236, -8.7072) -> (49.3236, -4.3826) projected
  line L53 (49.3236, -4.3826) -> (50.8236, -3.5166) projected
  line L54 (50.8236, -3.5166) -> (50.8236, 1.1022) projected
  line L55 (50.8236, 1.1022) -> (46.8236, 3.4116) projected
  line L56 (46.8236, 3.4116) -> (42.8236, 1.1022) projected
  line L57 (42.8236, 1.1022) -> (42.8236, -3.5166) projected
  line L58 (42.8236, -3.5166) -> (44.3236, -4.3826) projected
  line L59 (44.3236, -4.3826) -> (44.3236, -8.7072) projected
  line L60 (44.3236, -8.7072) -> (39.8236, -8.7072) projected
  line L61 (39.8236, -8.7072) -> (39.8236, -46.2472) projected
  line L62 (39.8236, -46.2472) -> (2.2836, -46.2472) projected
  line L63 (2.2836, -46.2472) -> (2.2836, -50.7472) projected
  line L64 (2.2836, -50.7472) -> (6.6082, -50.7472) projected
  line L65 (6.6082, -50.7472) -> (7.4742, -49.2472) projected
  line L66 (7.4742, -49.2472) -> (12.093, -49.2472) projected
  line L67 (12.093, -49.2472) -> (14.4024, -53.2472) projected
  line L68 (14.4024, -53.2472) -> (12.093, -57.2472) projected
  line L69 (12.093, -57.2472) -> (7.4742, -57.2472) projected
  line L70 (7.4742, -57.2472) -> (6.6082, -55.7472) projected
  line L71 (6.6082, -55.7472) -> (2.2836, -55.7472) projected
  line L72 (2.2836, -55.7472) -> (2.2836, -60.2472) projected
  line L73 (2.2836, -60.2472) -> (6.2836, -60.2472) projected
  line L74 (6.2836, -60.2472) -> (-8.7164, -82.1695) projected
  line L75 (-8.7164, -93.8615) -> (14.2836, -60.2472) projected
  line L76 (14.2836, -60.2472) -> (43.9241, -60.2472) projected
  line L77 (43.9241, -60.2472) -> (83.3844, -99.7074) projected
  line L78 (83.3844, -99.7074) -> (-8.7164, -99.7074) projected
  line L79 (-8.7164, -99.7074) -> (-8.7164, -93.8615) projected
  line L80 (53.8236, -20.6477) -> (87.2156, 2.2928) projected
  line L81 (87.2156, 2.2928) -> (93.2839, 2.2928) projected
  line L82 (93.2839, 2.2928) -> (93.2839, -89.8079) projected
  line L83 (93.2839, -89.8079) -> (53.8236, -50.3477) projected
  line L84 (53.8236, -50.3477) -> (53.8236, -20.6477) projected
  line L85 (-12.5976, -120.7074) -> (121.4113, -120.7074)
  line L86 (114.2839, 30.4116) -> (114.2839, -120.7074)
  line L87 (-24.7164, -127.7074) -> (114.2839, -127.7074)
  line L88 (44.7837, -127.7074) -> (44.7837, -115.891)
  circle A8 centre (44.7837, -120.7074) radius 2
  circle A9 centre (44.7837, -120.7074) radius 3.5412
  circle A10 centre (39.1837, -120.7074) radius 0.85
  line L89 (39.1837, -119.8574) -> (41.3461, -119.8574)
  line L90 (39.1837, -121.5574) -> (41.3461, -121.5574)
  line L91 (46.3837, -119.5074) -> (48.1154, -119.5074)
  line L92 (46.3837, -121.9074) -> (48.1154, -121.9074)
  line L93 (121.4113, 18.2928) -> (121.4113, -120.7074)
  line L94 (121.4113, -51.2073) -> (114.2839, -51.2073)
  line L95 (93.2839, -106.7074) -> (100.3476, -99.6437)
  line L96 (96.8157, -103.1756) -> (114.2839, -120.7074)
  line L97 (114.2839, -120.7074) -> (96.8157, -103.1756)
  line L98 (105.5498, -111.9415) -> (102.8506, -114.6308)
  point P0 (0, 0)
  point P1 (113.4338, -56.8046)
  point P2 (115.1339, -56.8056)
  point P3 (102.193, -107.3826)
  point P4 (100.9902, -108.584)
  point P5 (39.1865, -119.8574)
  point P6 (39.1855, -121.5574)
  constraints: 44 end point, 11 coincident, 9 centre point, 6 parallel, 6 point on line, 4 midpoint, 4 perpendicular, 3 vertical, 1 other
extrude "Vysunutí5" cut sketch "Náčrt3" against normal blind 4 contours L94 A1 L86 A0 | A0 L3 A1 L94 | L86 A1 L2 A0 | L86 A2 L0 A1 | A1 L1 A2 L86 | L86 A2 | A2 L86 | L91 A8 L88 A9 | A9 L88 A8 L92 | A4 L98 A3 L7 | L6 A3 L96 A4 | A9 L85 A8 L88 | L88 A8 L85 A9 | A4 L96 A3 L98 | L90 A10 L85 A9 | A9 L85 A10 L89 | L5 A5 L96 A4 | A4 L96 A5 L4 | A10 L85 | A10 L85 | A5 L96 | A5 L96 picked at (112.8391, -48.5747) picked at (108.5449, -111.6668)
